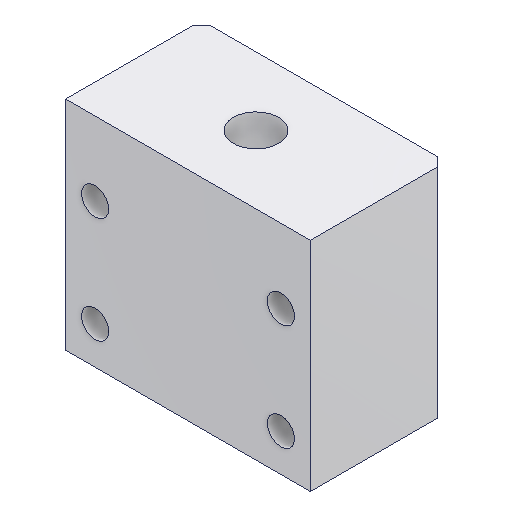
# Autodesk Inventor part: 3DP_ABS_Y_Axis_Tenioning_System_C_Sec_Filler
Saved by Autodesk Inventor 2026.1 (Build 301233000, 233)
## iProperties
Created: 2017-08-27
Part Number: 3DP_ABS_Y_Axis_Tenioning_System_C_Sec_Filler
Material: Ogólny
Document SubType Name: Modeling
Designer: Andrzej
Density: 1 g/cm^3
Appearance: PTFE
Author: Andrzej
Autodesk Inventor part; units mm, degrees
ref_plane "YZ Plane" through (0, 0, 0) normal (1, 0, 0) x (0, 1, 0)
ref_plane "XZ Plane" through (0, 0, 0) normal (0, 1, 0) x (-1, 0, 0)
ref_plane "XY Plane" through (0, 0, 0) normal (0, 0, 1) x (1, 0, 0)
sketch "Szkic1" plane through (0, 0, 0) normal (0, 0, 1) x (1, 0, 0)
  line L0 (27, 15) -> (0, 15)
  line L1 (0, 0) -> (0, 15)
  line L2 (27, 0) -> (0, 0)
  line L3 (27, 0) -> (27, 15)
  circle A0 centre (13.5, 7.5) radius 2.5
  point P0 (27, 22.2042)
  dimension "d0" = 27
  dimension "d1" = 15
  dimension "d2" = 7.5
  dimension "d3" = 13.5
  constraints: 8 end point, 1 centre point
  measures "d0" distance of L0.start L0.end
  measures "d1" distance of L2.start L0.start
  measures "d2" distance from line of L0 A0.centre
  measures "d3" distance from line of L3 A0.centre
extrude "Wyciągnięcie proste1" add sketch "Szkic1" along normal blind 24
chamfer "Faza1" distance 1 angle 45 2 edges at (27, 15, 12) (0, 15, 12)
sketch "Szkic4" plane through (0, 0, 0) normal (0, -1, 0) x (1, 0, 0)
  line L0 (0, 0) -> (27, 0) projected
  line L1 (27, 0) -> (27, 24) projected
  line L2 (0, 24) -> (27, 24) projected
  line L3 (0, 0) -> (0, 24) projected
  point P0 (3.25, 4.15)
  point P1 (3.25, 15.85)
  point P2 (23.75, 4.15)
  point P3 (23.75, 15.85)
  dimension "d9" = 20.5
  dimension "d10" = 11.7
  dimension "d11" = 4.15
  dimension "d12" = 27
  dimension "d13" = 3.25
  constraints: 2 horizontal alignment, 2 vertical alignment
  measures "d9" distance of point (23.75, 4.15) point (3.25, 4.15)
  measures "d10" distance of point (3.25, 4.15) point (3.25, 15.85)
  measures "d11" distance from line of L0 point (3.25, 4.15)
  measures "d12" distance of L0.start L0.end
  measures "d13" distance from line of L3 point (3.25, 4.15)
hole "Otwór1" at (3.25, 0, 4.15) at (3.25, 0, 15.85) at (23.75, 0, 4.15) at (23.75, 0, 15.85) direction (0, 1, 0) diameter 3 end through all
equation "\"d13\" = -0.5 * d9 + 0.5 * d12"
